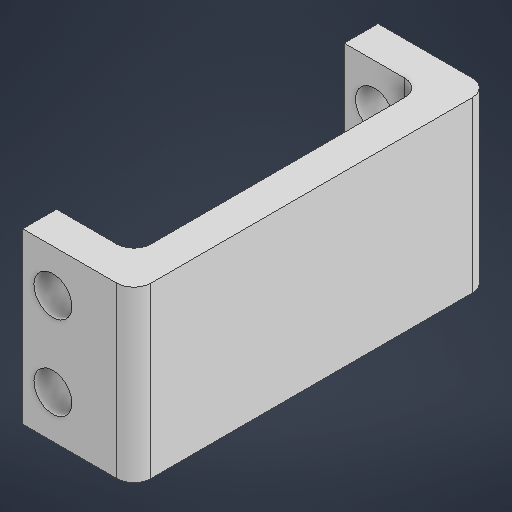
# Autodesk Inventor part: крепл сервы на пуляло
Saved by Autodesk Inventor 2026.2 (Build 302298000, 298)
## iProperties
Created: 2025-12-24
Part Number: крепл сервы на пуляло
Material: Типовые
Document SubType Name: Modeling
Designer: Phantom
Density: 1 g/cm^3
Appearance: По умолчанию
Author: Phantom
Autodesk Inventor part; units mm, degrees
ref_plane "YZ Plane" through (0, 0, 0) normal (1, 0, 0) x (0, 1, 0)
ref_plane "XZ Plane" through (0, 0, 0) normal (0, 1, 0) x (-1, 0, 0)
ref_plane "XY Plane" through (0, 0, 0) normal (0, 0, 1) x (1, 0, 0)
sketch "Эскиз1" plane through (0, 0, 0) normal (0, 0, 1) x (1, 0, 0)
  line L0 (21.232, 7.9335) -> (21.232, 9.4835)
  arc A0 (21.232, 9.4835) -> (19.732, 10.9835) centre (19.732, 9.4835) ccw
  line L1 (19.732, 10.9835) -> (-31.568, 10.9835)
  line L2 (-31.568, -9.0165) -> (19.732, -9.0165)
  arc A1 (19.732, -9.0165) -> (21.232, -7.5165) centre (19.732, -7.5165) ccw
  line L3 (21.232, -7.5165) -> (21.232, -5.9665)
  line L4 (21.232, -5.9665) -> (19.1128, -5.9665)
  arc A2 (19.1128, -1.9665) -> (19.1128, -5.9665) centre (18.082, -3.9665) ccw
  line L5 (19.1128, -1.9665) -> (21.232, -1.9665)
  line L6 (21.232, -1.9665) -> (21.232, 3.9335)
  line L7 (21.232, 3.9335) -> (19.1128, 3.9335)
  arc A3 (19.1128, 7.9335) -> (19.1128, 3.9335) centre (18.082, 5.9335) ccw
  line L8 (19.1128, 7.9335) -> (21.232, 7.9335)
  line L9 (-24.768, -8.9965) -> (13.532, -8.9965)
  line L10 (13.532, 10.9635) -> (-24.768, 10.9635)
  arc A4 (14.512, 9.9835) -> (13.532, 10.9635) centre (13.532, 9.9835) ccw
  line L11 (14.512, -8.0165) -> (14.512, 9.9835)
  arc A5 (13.532, -8.9965) -> (14.512, -8.0165) centre (13.532, -8.0165) ccw
  line L12 (14.512, 9.9835) -> (14.512, 13.5721)
  line L13 (21.652, -9.0165) -> (14.512, -9.0165)
  line L14 (14.512, -9.0165) -> (14.512, 10.9835)
  line L15 (14.512, 10.9835) -> (21.652, 10.9835)
  line L16 (21.652, 10.9835) -> (21.652, -9.0165)
  line L17 (21.652, -9.0165) -> (14.512, 10.9835) construction
  line L18 (14.512, -9.0165) -> (21.652, 10.9835) construction
  circle A6 centre (18.082, 5.9335) radius 2.25
  circle A7 centre (18.082, -3.9665) radius 2.25
  line L19 (21.652, 10.9835) -> (23.652, 10.9835)
  line L20 (23.652, 10.9835) -> (23.652, -9.0165)
  line L21 (23.652, -9.0165) -> (21.652, -9.0165)
  line L22 (21.652, -9.0165) -> (21.652, 10.9835)
  point P0 (0, 0)
  point P1 (-5.918, 0.9835)
  point P2 (18.082, 0.9835)
  point P3 (19.1128, -5.9665)
  point P4 (19.732, -9.0165)
  dimension "d2" = 2
  constraints: 46 end point, 12 point on circle, 8 centre point, 4 parallel, 2 coincident, 2 concentric, 2 horizontal, 2 midpoint, 2 perpendicular, 2 point on line, 1 vertical
  measures "d2" distance of L20.end L21.end
extrude "Выдавливание1" add sketch "Эскиз1" along normal blind 4 contours L8 A3 L7 L6 L5 A2 L4 L3 A1 L2 L14 L11 L12 L1 A0 L0 | L0 A0 L15 L16 L13 A1 L3 L4 A7 L5 L6 L7 A6 L8 | L19 L20 L21 L16
sketch "Эскиз2" plane through (0, 0, 4) normal (0, 0, 1) x (1, 0, 0)
  line L0 (23.652, 10.9835) -> (14.512, 10.9835) projected
  line L1 (14.512, 10.9835) -> (14.512, -9.0165) projected
  line L2 (14.512, -9.0165) -> (23.652, -9.0165) projected
  line L3 (23.652, -9.0165) -> (23.652, 10.9835) projected
  circle A0 centre (18.082, -3.9665) radius 2.25 projected
  circle A1 centre (18.082, 5.9335) radius 2.25 projected
  line L4 (23.652, 10.9835) -> (27.652, 10.9835)
  line L5 (27.652, 10.9835) -> (27.652, -9.0165)
  line L6 (27.652, -9.0165) -> (23.652, -9.0165)
  line L7 (23.652, -9.0165) -> (23.652, 10.9835)
  point P0 (0, 0)
  dimension "d3" = 4
  constraints: 8 end point, 2 parallel, 1 horizontal, 1 perpendicular
  measures "d3" distance of L5.end L6.end
extrude "Выдавливание2" add sketch "Эскиз2" against normal blind 42 contours L4 L5 L6 L3
sketch "Эскиз3" plane through (0, 0, -38) normal (0, 0, -1) x (-1, 0, 0)
  line L0 (-23.652, 10.9835) -> (-14.512, 10.9835) projected
  line L1 (-23.652, -9.0165) -> (-23.652, 10.9835) projected
  line L2 (-14.512, -9.0165) -> (-23.652, -9.0165) projected
  line L3 (-14.512, 10.9835) -> (-14.512, -9.0165) projected
  circle A0 centre (-18.082, -3.9665) radius 2.25 projected
  circle A1 centre (-18.082, 5.9335) radius 2.25 projected
  point P0 (0, 0)
extrude "Выдавливание3" add sketch "Эскиз3" against normal blind 4
fillet "Сопряжение1" radius 2 4 edges at (23.652, 0.9835, 0) (23.652, 0.9835, -34) (27.652, 0.9835, -38) (27.652, 0.9835, 4)
